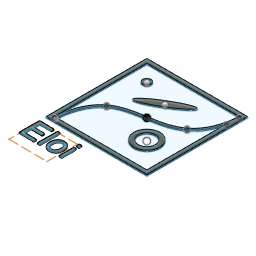
2023_05_26_3D Print on T Shirt v1 (Autodesk Fusion 360 design; units mm, degrees)
Autodesk Fusion 360 part; units mm, degrees
sketch "Esquisse1" plane through (0, 0, 0) normal (0, 0, 1) x (1, 0, 0)
  line L0 (-25, 25) -> (25, 25)
  line L1 (25, 25) -> (25, -25)
  line L2 (25, -25) -> (-25, -25)
  line L3 (-25, -25) -> (-25, 25)
  line L4 (-23, -23) -> (-23, 23)
  line L5 (-23, 23) -> (23, 23)
  line L6 (23, 16.6659) -> (23, -23)
  line L7 (23, -23) -> (-21.9957, -23)
  spline S0 degree 5 poles (-23, -23) (-22.9089, -22.0117) (-22.6865, -20.093) (-22.2316, -17.3883) (-21.382, -14.1303) (-19.9116, -10.6425) (-18.034, -7.7377) (-15.7596, -5.4009) (-13.1136, -3.5964) (-10.1426, -2.2571) (-6.9125, -1.2889) (-3.5023, -0.5785) (0, 0) (3.5023, 0.5785) (6.9125, 1.2889) (10.1426, 2.2571) (13.1136, 3.5964) (15.7596, 5.4009) (18.034, 7.7377) (19.9116, 10.6425) (21.382, 14.1303) (22.2316, 17.3883) (22.6865, 20.093) (22.9089, 22.0117) (23, 23) knots 0 0 0 0 0 0 0.05 0.1 0.15 0.2 0.25 0.3 0.35 0.4 0.45 0.5 0.55 0.6 0.65 0.7 0.75 0.8 0.85 0.9 0.95 1 1 1 1 1 1
  spline S1 degree 3 poles (-22.0042, -23.0917) (-21.4648, -17.2374) (-20.058, -12.7108) (-17.8645, -9.4748) (-15.8058, -6.4378) (-13.0401, -4.5207) (-9.6673, -3.2638) (-5.6169, -1.7543) (-0.721, -1.2254) (4.0189, -0.3032) (7.7314, 0.4191) (11.3416, 1.4225) (14.3899, 3.3598) (17.2674, 5.1884) (19.6042, 7.8592) (21.2274, 11.4106) (21.9507, 12.993) (22.5399, 14.7452) (23, 16.6659) knots 0 0 0 0 0.181061 0.181061 0.181061 0.350992 0.350992 0.350992 0.555061 0.555061 0.555061 0.714901 0.714901 0.714901 0.865783 0.865783 0.865783 0.933015 0.933015 0.933015 0.933015
  circle A0 centre (-15, 15) radius 2
  circle A1 centre (10, -10) radius 4.2426
  circle A2 centre (10, -10) radius 6.4031
  ellipse E0 centre (-1, 10) end of major axis (9, 16) minor radius 1.8819
  line L8 (-11, 4) -> (9, 16)
  line L9 (-0.0318, 8.3863) -> (-1.9682, 11.6137)
  line L10 (-25.0792, -43.4247) -> (-6.0774, -43.6428) construction
  line L11 (-6.0774, -43.6428) -> (-5.905, -28.6163) construction
  line L12 (-5.905, -28.6163) -> (-24.9068, -28.3983) construction
  line L13 (-24.9068, -28.3983) -> (-25.0792, -43.4247) construction
  point P0 (-15, -5)
  point P1 (15, 5)
  dimension "d5" = 10
  text T0 "Eloi" font "Arial" height 10 align left top in box 19.003 x 15.0274 at (-25.0792, -43.4247) x (0.999934, -0.011474) y (0.011474, 0.999934) spacing 1 kerned
  constraint horizontal L0
  constraint vertical L1
  constraint horizontal L2
  constraint vertical L3
  constraint parallel L3 L4
  constraint parallel L0 L5
  constraint parallel L1 L6
  constraint parallel L2 L7
  constraint coincident S1 L7.end
  constraint concentric A1 A2
  constraint coincident E0 L8.start
  constraint coincident E0 L8.end
  constraint coincident E0 L9.start
  constraint coincident E0 L9.end
extrude "Extrusion1" add sketch "Esquisse1" sketch "Esquisse1" along normal blind 0.6 of sketch 2 text T0 makes body 1 at (24.3333, 5.5553, 0) makes body 2 at (-15.0589, -35.1784, 0) makes body 3 at (-12.7368, -34.4156, 0) makes body 4 at (-14.5843, 14.9427, 0) makes body 5 at (2.164, 11.2161, 0) makes body 6 at (15.6433, -10.5289, 0) makes body 7 at (-4.0867, -29.5786, 0) makes body 8 at (-4.5445, -33.8028, 0) makes body 9 at (-24.5246, -33.5417, 0)
